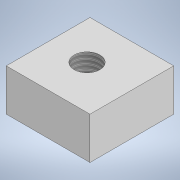
# Autodesk Inventor part: testThread
Saved by Autodesk Inventor 2021 (Build 250183000, 183)
## iProperties
Created: 2020-04-13
Part Number: testThread
Material: Generic
Document SubType Name: Modeling
Designer: robst
Density: 1 g/cm^3
Appearance: Default
Author: robst
Autodesk Inventor part; units mm, degrees
ref_plane "YZ Plane" through (0, 0, 0) normal (1, 0, 0) x (0, 1, 0)
ref_plane "XZ Plane" through (0, 0, 0) normal (0, 1, 0) x (-1, 0, 0)
ref_plane "XY Plane" through (0, 0, 0) normal (0, 0, 1) x (1, 0, 0)
sketch "Sketch1" plane through (0, 0, 0) normal (0, 1, 0) x (-1, 0, 0)
  line L0 (-12.7, 12.7) -> (-12.7, -12.7)
  line L1 (-12.7, -12.7) -> (12.7, -12.7)
  line L2 (12.7, -12.7) -> (12.7, 12.7)
  line L3 (12.7, 12.7) -> (-12.7, 12.7)
  line L4 (-12.7, 12.7) -> (12.7, -12.7) construction
  line L5 (-12.7, -12.7) -> (12.7, 12.7) construction
  point P0 (0, 0)
  dimension "d0" = 25.4
  constraints: 12 end point, 2 midpoint, 2 parallel, 2 perpendicular, 1 vertical
  measures "d0" distance of L0.start L0.end
extrude "Extrusion1" add sketch "Sketch1" against normal blind 12.7
sketch "Sketch3" plane through (0, 0, 0) normal (0, 1, 0) x (1, 0, 0)
  point P0 (0, 0)
  point P1 (-1.3731, 0.4703)
hole "Hole2" at (-1.3731, 0, -0.4703) direction (0, -1, 0) diameter 7.7978 end through all
thread "Thread2" size "5/16-18 UNC" class "2B" standard "ANSI Unified Screw Threads" full length
body "Solid1"
